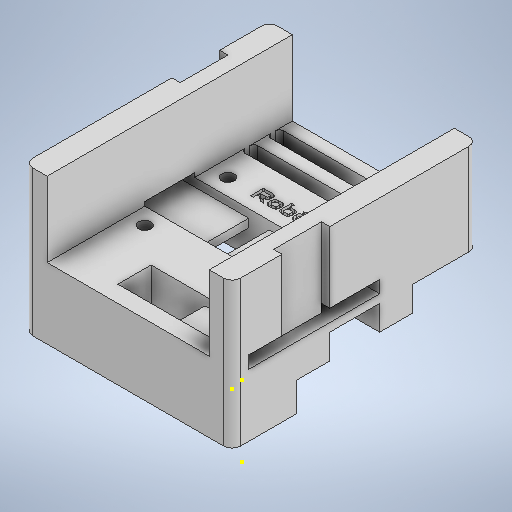
# Autodesk Inventor part: CaseInterno
Saved by Autodesk Inventor 2025.2 (Build 292293000, 293)
## iProperties
Created: 2025-03-20
Part Number: CaseInterno
Material: Genérico
Document SubType Name: Modeling
Designer: miche
Density: 1 g/cm^3
Appearance: Padrão
Author: miche
Autodesk Inventor part; units mm, degrees
ref_plane "YZ Plane" through (0, 0, 0) normal (1, 0, 0) x (0, 1, 0)
ref_plane "XZ Plane" through (0, 0, 0) normal (0, 1, 0) x (-1, 0, 0)
ref_plane "XY Plane" through (0, 0, 0) normal (0, 0, 1) x (1, 0, 0)
sketch "Esboço1" plane through (0, 0, 0) normal (0, 1, 0) x (-1, 0, 0)
  line L0 (5, 0) -> (50, 0)
  line L1 (55, -5) -> (55, -54)
  line L2 (50, -59) -> (5, -59)
  line L3 (0, -54) -> (0, -5)
  arc A0 (50, -59) -> (55, -54) centre (50, -54) ccw
  arc A1 (0, -54) -> (5, -59) centre (5, -54) ccw
  arc A2 (5, 0) -> (0, -5) centre (5, -5) ccw
  arc A3 (55, -5) -> (50, 0) centre (50, -5) ccw
  point P0 (0, 0)
  point P1 (55, -59)
  point P2 (55, 0)
  point P3 (0, -59)
  dimension "d0" = 55
  dimension "d1" = 59
  dimension "d2" = 5
  constraints: 8 end point, 8 point on circle, 8 point on line, 8 tangent, 4 centre point, 3 equal radius, 2 parallel, 1 horizontal, 1 perpendicular
  measures "d0" distance of point (55, -59) point (0, -59)
  measures "d1" distance of point (55, 0) point (55, -59)
  measures "d2" radius of A0
extrude "Extrusão1" add sketch "Esboço1" along normal blind 5
sketch "Esboço2" plane through (0, 0, 0) normal (0, -1, 0) x (1, 0, 0)
  line L0 (-5, -59) -> (-50, -59) projected
  line L1 (-50, -59) -> (-55, -59)
  arc A0 (-55, -54) -> (-50, -59) centre (-50, -54) ccw projected
  line L2 (-55, -59) -> (-55, -43.5)
  line L3 (-55, -54) -> (-55, -5) projected
  line L4 (-55, -5) -> (-55, 0)
  line L5 (-55, 0) -> (-50, 0)
  line L6 (-55, 0) -> (-55, -15.5)
  line L7 (0, -5) -> (0, -54) projected
  line L8 (-55, -43.5) -> (0, -43.5)
  line L9 (0, -43.5) -> (0, -35.5)
  line L10 (0, -35.5) -> (-55, -35.5)
  line L11 (-55, -35.5) -> (-55, -43.5)
  line L12 (-55, -15.5) -> (0, -15.5)
  line L13 (0, -15.5) -> (0, -23.5)
  line L14 (0, -23.5) -> (-55, -23.5)
  line L15 (-55, -23.5) -> (-55, -15.5)
  line L16 (-55, -35.5) -> (-55, -23.5)
  line L17 (0, -35.5) -> (0, -23.5)
  point P0 (0, 0)
  dimension "d5" = 15.5
  dimension "d6" = 15.5
  dimension "d7" = 8
  dimension "d8" = 8
  constraints: 30 end point, 4 parallel, 4 point on line, 3 horizontal, 3 perpendicular, 1 collinear, 1 tangent, 1 vertical
  measures "d5" distance of L1.end L2.end
  measures "d6" distance of L4.end L6.end
  measures "d7" distance of L9.end L8.end
  measures "d8" distance of L12.end L13.end
extrude "Extrusão2" add sketch "Esboço2" along normal blind 6 contours L3 L10 L7 L8 | L3 L12 L7 L14
sketch "Esboço3" plane through (0, -6, 0) normal (0, -1, 0) x (1, 0, 0)
  line L0 (-55, -43.5) -> (0, -43.5) projected
  line L1 (-55, -35.5) -> (0, -35.5) projected
  line L2 (0, -43.5) -> (-24, -43.5)
  line L3 (-24, -43.5) -> (-24, -35.5)
  line L4 (-24, -35.5) -> (0, -35.5)
  line L5 (0, -35.5) -> (0, -43.5)
  line L6 (-55, -35.5) -> (-55, -43.5) projected
  line L7 (-55, -43.5) -> (-31, -43.5)
  line L8 (-31, -43.5) -> (-31, -35.5)
  line L9 (-31, -35.5) -> (-55, -35.5)
  line L10 (-55, -35.5) -> (-55, -43.5)
  line L11 (-24, -43.5) -> (-31, -43.5)
  line L12 (-31, -43.5) -> (-31, -35.5)
  line L13 (-31, -35.5) -> (-24, -35.5)
  line L14 (-24, -35.5) -> (-24, -43.5)
  line L15 (-55, -15.5) -> (0, -15.5) projected
  line L16 (0, -23.5) -> (-55, -23.5) projected
  line L17 (0, -15.5) -> (-24, -15.5)
  line L18 (-24, -15.5) -> (-24, -23.5)
  line L19 (-24, -23.5) -> (0, -23.5)
  line L20 (0, -23.5) -> (0, -15.5)
  line L21 (-24, -23.5) -> (-31, -23.5)
  line L22 (-31, -23.5) -> (-31, -15.5)
  line L23 (-31, -15.5) -> (-24, -15.5)
  line L24 (-24, -15.5) -> (-24, -23.5)
  point P0 (0, 0)
  constraints: 40 end point, 10 parallel, 6 point on line, 5 horizontal, 5 perpendicular
extrude "Extrusão3" add sketch "Esboço3" along normal blind 16 contours L8 L1 L3 L0 | L15 L18 L16 L22
sketch "Esboço4" plane through (0, -6, 0) normal (0, -1, 0) x (1, 0, 0)
  line L0 (0, -43.5) -> (-55, -43.5) projected
  line L1 (0, -43.5) -> (-12, -43.5)
  line L2 (-12, -43.5) -> (-12, -39.5)
  line L3 (-55, -43.5) -> (-43, -43.5)
  line L4 (-55, -43.5) -> (-31, -43.5) projected
  line L5 (-43, -43.5) -> (-43, -39.5)
  line L6 (-55, -15.5) -> (0, -15.5) projected
  line L7 (0, -15.5) -> (-12, -15.5)
  line L8 (-12, -15.5) -> (-12, -19.5)
  line L9 (-55, -15.5) -> (-43, -15.5)
  line L10 (-55, -15.5) -> (-43, -15.5)
  line L11 (-43, -15.5) -> (-43, -19.5)
  circle A0 centre (-12, -39.5) radius 1.5
  circle A1 centre (-12, -19.5) radius 1.5
  circle A2 centre (-43, -39.5) radius 1.5
  circle A3 centre (-43, -19.5) radius 1.5
  point P0 (0, 0)
  dimension "d13" = 4
  dimension "d14" = 12
  dimension "d15" = 4
  dimension "d16" = 12
  dimension "d17" = 4
  dimension "d18" = 12
  dimension "d19" = 4
  dimension "d20" = 3
  dimension "d21" = 3
  dimension "d22" = 3
  dimension "d23" = 3
  constraints: 18 end point, 4 centre point, 4 coincident, 3 perpendicular, 3 point on line, 1 collinear, 1 midpoint, 1 vertical
  measures "d13" distance of L1.end L2.end
  measures "d14" distance of L0.end L3.end
  measures "d15" distance of L3.end L5.end
  measures "d16" distance of L6.end L7.end
  measures "d17" distance of L7.end L8.end
  measures "d18" distance of L6.start L9.end
  measures "d19" distance of L9.end L11.end
  measures "d20" diameter of A0
  measures "d21" diameter of A1
  measures "d22" diameter of A2
  measures "d23" diameter of A3
extrude "Extrusão4" cut sketch "Esboço4" against normal blind 11
thread "Rosca1" size "M3x0.5" class "6H" standard "ANSI Metric M Profile" length 11
thread "Rosca2" size "M3x0.5" class "6H" standard "ANSI Metric M Profile" full length
thread "Rosca3" size "M3x0.5" class "6H" standard "ANSI Metric M Profile" full length
thread "Rosca4" size "M3x0.5" class "6H" standard "ANSI Metric M Profile" full length
thread "Rosca5" size "M3x0.5" class "6H" standard "ANSI Metric M Profile" length 11
thread "Rosca6" size "M3x0.5" class "6H" standard "ANSI Metric M Profile" length 11
thread "Rosca7" size "M3x0.5" class "6H" standard "ANSI Metric M Profile" length 11
sketch "Esboço7" plane through (0, 0, 0) normal (0, -1, 0) x (1, 0, 0)
  line L0 (-55, -35.5) -> (0, -35.5) projected
  line L1 (0, -35.5) -> (-24, -35.5)
  line L2 (-31, -23.5) -> (-31, -15.5) projected
  line L3 (-24, -35.5) -> (-31, -35.5)
  line L4 (-31, -35.5) -> (-31, -23.5)
  line L5 (-31, -23.5) -> (-24, -23.5)
  line L6 (-24, -23.5) -> (-24, -35.5)
  point P0 (0, 0)
  constraints: 10 end point, 2 parallel, 1 horizontal, 1 perpendicular, 1 point on line
extrude "Extrusão7" add sketch "Esboço7" along normal blind 6
sketch "Esboço9" plane through (0, 0, 0) normal (0, -1, 0) x (1, 0, 0)
  line L0 (0, -5) -> (0, -15.5) projected
  line L1 (0, -15.5) -> (0, -5)
  line L2 (-50, 0) -> (-5, 0) projected
  arc A0 (0, -5) -> (-5, 0) centre (-5, -5) ccw
  line L3 (-55, -15.5) -> (0, -15.5) projected
  line L4 (-55, -15.5) -> (-55, -5)
  arc A1 (-50, 0) -> (-55, -5) centre (-50, -5) ccw projected
  line L5 (-5, 0) -> (-50, 0)
  arc A2 (-50, 0) -> (-55, -5) centre (-50, -5) ccw
  point P0 (0, 0)
  constraints: 6 end point, 4 point on circle, 2 centre point, 2 tangent, 1 collinear, 1 horizontal
sketch "Esboço10" plane through (0, 0, 0) normal (0, -1, 0) x (1, 0, 0)
  line L0 (-24, -35.5) -> (-24, -23.5) projected
  line L1 (-24, -23.5) -> (0, -23.5) projected
  line L2 (-24, -35.5) -> (-21, -35.5)
  line L3 (-21, -35.5) -> (-21, -23.5)
  line L4 (-21, -23.5) -> (-24, -23.5)
  line L5 (-24, -23.5) -> (-24, -35.5)
  line L6 (-31, -23.5) -> (-31, -35.5) projected
  line L7 (-31, -35.5) -> (-34, -35.5)
  line L8 (-34, -35.5) -> (-34, -23.5)
  line L9 (-34, -23.5) -> (-31, -23.5)
  line L10 (-31, -23.5) -> (-31, -35.5)
  point P0 (0, 0)
  constraints: 16 end point, 4 parallel, 2 horizontal, 2 perpendicular, 2 point on line
extrude "Extrusão9" cut sketch "Esboço10" against normal through all
sketch "Esboço11" plane through (0, 5, 0) normal (0, 1, 0) x (1, 0, 0)
  line L0 (-34, 23.5) -> (-34, 35.5)
  line L1 (-24, 23.5) -> (-24, 35.5) projected
  line L2 (-31, 23.5) -> (-31, 35.5) projected
  line L3 (-24, 35.5) -> (-31, 35.5)
  line L4 (-31, 35.5) -> (-31, 23.5)
  line L5 (-31, 23.5) -> (-24, 23.5)
  line L6 (-24, 23.5) -> (-24, 35.5)
  line L7 (-21, 35.5) -> (0, 35.5) projected
  line L8 (0, 23.5) -> (-21, 23.5) projected
  line L9 (-21, 35.5) -> (-2, 35.5)
  line L10 (-2, 23.5) -> (-21, 23.5)
  line L11 (-21, 23.5) -> (-21, 35.5)
  line L12 (-2, 35.5) -> (0, 35.5)
  line L13 (0, 35.5) -> (0, 23.5)
  line L14 (0, 23.5) -> (-2, 23.5)
  line L15 (-2, 23.5) -> (-2, 35.5)
  point P0 (0, 0)
  constraints: 24 end point, 5 parallel, 3 horizontal, 2 perpendicular, 1 point on line
extrude "Extrusão10" cut sketch "Esboço11" against normal blind 2
extrude "Extrusão11" add sketch "Esboço9" along normal blind 13
sketch "Esboço12" plane through (0, -13, 0) normal (0, -1, 0) x (1, 0, 0)
  line L0 (-9.5, 0) -> (-5, 0) projected
  line L1 (-5, 0) -> (-5, -15.5)
  line L2 (-5, -23.5) -> (-5, 0) projected
  line L3 (0, -15.5) -> (-24, -15.5) projected
  line L4 (0, -15.5) -> (-55, -15.5)
  line L5 (0, -15.5) -> (-20, -15.5)
  line L6 (-20, -15.5) -> (-12.7, -15.5) construction
  line L7 (-20, -13) -> (-35, -13)
  line L8 (-35, -13) -> (-35, -3)
  line L9 (-35, -3) -> (-20, -3)
  line L10 (-20, -3) -> (-20, -13)
  point P0 (0, 0)
  constraints: 16 end point, 3 horizontal, 2 parallel, 2 point on line, 1 perpendicular
extrude "Extrusão12" cut sketch "Esboço12" against normal blind 1
sketch "Esboço13" plane through (0, -12, 0) normal (0, -1, 0) x (1, 0, 0)
  line L0 (-35, -13) -> (-35, -3) projected
  line L1 (-35, -3) -> (-34, -3)
  line L2 (-35, -3) -> (-20, -3) projected
  line L3 (-34, -3) -> (-34, -4)
  line L4 (-34, -4) -> (-21, -4)
  line L5 (-21, -4) -> (-21, -12)
  line L6 (-21, -12) -> (-34, -12)
  line L7 (-34, -12) -> (-34, -4)
  point P0 (0, 0)
  constraints: 12 end point, 2 parallel, 1 horizontal, 1 perpendicular, 1 point on line, 1 vertical
extrude "Extrusão13" cut sketch "Esboço13" against normal blind 16
sketch "Esboço14" plane through (0, 5, 0) normal (0, 1, 0) x (1, 0, 0)
  line L0 (-21, 12) -> (-34, 12) projected
  line L1 (-34, 12) -> (-21, 12)
  line L2 (-21, 12) -> (-21, 4)
  line L3 (-21, 4) -> (-34, 4)
  line L4 (-34, 4) -> (-34, 12)
  line L5 (-21, 12) -> (-2, 12)
  line L6 (-2, 4) -> (-21, 4)
  line L7 (-21, 4) -> (-21, 12) projected
  line L8 (-21, 12) -> (-21, 4)
  line L9 (-2, 12) -> (0, 12)
  line L10 (0, 12) -> (0, 4)
  line L11 (0, 4) -> (-2, 4)
  line L12 (-2, 4) -> (-2, 12)
  point P0 (0, 0)
  constraints: 22 end point, 4 perpendicular, 3 equal length, 1 horizontal, 1 point on line, 1 vertical
extrude "Extrusão14" cut sketch "Esboço14" against normal blind 2
sketch "Esboço16" plane through (0, 5, 0) normal (0, 1, 0) x (1, 0, 0)
  arc A0 (-50, 59) -> (-55, 54) centre (-50, 54) ccw projected
  line L0 (-55, 54) -> (-55, 5) projected
  line L1 (-55, 54) -> (-55, 5)
  line L2 (-55, 5) -> (-47, 5)
  line L3 (-47, 5) -> (-47, 54)
  line L4 (-47, 54) -> (-55, 54)
  line L5 (-47, 5) -> (-47, 0)
  line L6 (-47, 54) -> (-47, 59)
  line L7 (-5, 59) -> (-50, 59) projected
  arc A1 (-50, 59) -> (-55, 54) centre (-50, 54) ccw
  arc A2 (-55, 5) -> (-50, 0) centre (-50, 5) ccw
  arc A3 (0, 54) -> (-5, 59) centre (-5, 54) ccw projected
  arc A4 (0, 54) -> (-5, 59) centre (-5, 54) ccw
  arc A5 (-5, 0) -> (0, 5) centre (-5, 5) ccw projected
  arc A6 (-5, 0) -> (0, 5) centre (-5, 5) ccw
  line L8 (0, 43.5) -> (0, 54) projected
  line L9 (0, 54) -> (0, 5)
  line L10 (0, 54) -> (-8, 54)
  line L11 (-8, 54) -> (-8, 59)
  line L12 (-8, 54) -> (-8, 4)
  line L13 (-0.101, 4) -> (-21, 4) projected
  line L14 (-5, 0) -> (-50, 0) projected
  line L15 (-8, 0) -> (-5, 0)
  line L16 (-8, 4) -> (-8, 0)
  point P0 (0, 0)
  constraints: 24 end point, 8 point on circle, 6 point on line, 5 tangent, 4 centre point, 3 collinear, 3 perpendicular, 3 vertical, 1 horizontal
extrude "Extrusão15" add sketch "Esboço16" along normal blind 17 contours L7 L6 L4 A0 | L4 L3 L2 L0 | L2 L5 L14 A2 | L7 A3 L10 L11 | L10 L8 L9 A5 L13 L12 | L13 A5 L14 L16
sketch "Esboço20" plane through (0, 0, 0) normal (0, -1, 0) x (1, 0, 0)
  arc A0 (-5, -59) -> (0, -54) centre (-5, -54) ccw projected
  line L0 (-9, -55.9) -> (-46, -55.9)
  line L1 (-8, -55.9) -> (-47, -55.9)
  line L2 (-47, -54.9) -> (-47, -53.8)
  line L3 (-46, -52.8) -> (-9, -52.8)
  line L4 (-8, -53.8) -> (-8, -54.9)
  line L5 (-8, -52.8) -> (-47, -52.8)
  line L6 (-47, -49.7) -> (-9, -49.7)
  line L7 (-8, -49.7) -> (-46, -49.7)
  line L8 (-47, -48.7) -> (-47, -47.6)
  line L9 (-46, -46.6) -> (-9, -46.6)
  line L10 (-8, -47.6) -> (-8, -48.7)
  arc A1 (-9, -55.9) -> (-8, -54.9) centre (-9, -54.9) ccw
  arc A2 (-8, -53.8) -> (-9, -52.8) centre (-9, -53.8) ccw
  arc A3 (-47, -54.9) -> (-46, -55.9) centre (-46, -54.9) ccw
  arc A4 (-46, -52.8) -> (-47, -53.8) centre (-46, -53.8) ccw
  arc A5 (-9, -49.7) -> (-8, -48.7) centre (-9, -48.7) ccw
  arc A6 (-8, -47.6) -> (-9, -46.6) centre (-9, -47.6) ccw
  arc A7 (-46, -46.6) -> (-47, -47.6) centre (-46, -47.6) ccw
  arc A8 (-47, -48.7) -> (-46, -49.7) centre (-46, -48.7) ccw
  point P0 (0, 0)
  dimension "d97" = 1
  constraints: 22 end point, 16 point on circle, 16 tangent, 8 centre point, 7 equal radius, 7 point on line, 5 parallel, 3 horizontal, 2 perpendicular
  measures "d97" radius of A1
extrude "Extrusão18" cut sketch "Esboço20" against normal through all
sketch "Esboço22" plane through (0, 5, 0) normal (0, 1, 0) x (1, 0, 0)
  line L0 (-39.1857, 44.1197) -> (-14.6747, 44.1197) construction
  line L1 (-14.6747, 44.1197) -> (-14.6747, 36.2889) construction
  line L2 (-14.6747, 36.2889) -> (-39.1857, 36.2889) construction
  line L3 (-39.1857, 36.2889) -> (-39.1857, 44.1197) construction
  spline S0 degree 2 poles (-33.3948, 40.4658) (-33.3948, 40.2734) (-33.4897, 39.97) (-33.6549, 39.7342) (-33.8663, 39.569) (-34.0993, 39.4633) (-34.335, 39.4145) (-34.3946, 39.4145) knots 0 0 0 1 2 3 4 5 6 6 6
  line L4 (-34.3946, 39.4145) -> (-33.2648, 38.4392)
  line L5 (-33.2648, 38.4392) -> (-34.1643, 38.4392)
  line L6 (-34.1643, 38.4392) -> (-35.2941, 39.4145)
  line L7 (-35.2941, 39.4145) -> (-35.7087, 39.4145)
  line L8 (-35.7087, 39.4145) -> (-35.7087, 40.0431)
  line L9 (-35.7087, 40.0431) -> (-34.438, 40.0431)
  spline S1 degree 2 poles (-34.438, 40.0431) (-34.3513, 40.0512) (-34.1941, 40.1136) (-34.0857, 40.2192) (-34.0234, 40.3682) (-34.0234, 40.4658) knots 0 0 0 1 2 3 4 4 4
  line L10 (-34.0234, 40.4658) -> (-34.0234, 40.8072)
  spline S2 degree 2 poles (-34.0234, 40.8072) (-34.0234, 40.8424) (-34.037, 40.8695) (-34.0532, 40.8803) (-34.083, 40.883) (-34.0966, 40.883) knots 0 0 0 1 2 3 4 4 4
  line L11 (-34.0966, 40.883) -> (-35.836, 40.883)
  line L12 (-35.836, 40.883) -> (-35.836, 38.4392)
  line L13 (-35.836, 38.4392) -> (-36.4673, 38.4392)
  line L14 (-36.4673, 38.4392) -> (-36.4673, 41.1946)
  spline S3 degree 2 poles (-36.4673, 41.1946) (-36.4673, 41.2623) (-36.4212, 41.3761) (-36.3345, 41.4628) (-36.218, 41.5116) (-36.1503, 41.5116) knots 0 0 0 1 2 3 4 4 4
  line L15 (-36.1503, 41.5116) -> (-34.0966, 41.5116)
  spline S4 degree 2 poles (-34.0966, 41.5116) (-33.9042, 41.5116) (-33.6333, 41.3707) (-33.468, 41.1594) (-33.3948, 40.9155) (-33.3948, 40.8099) knots 0 0 0 1 2 3 4 4 4
  line L16 (-33.3948, 40.8099) -> (-33.3948, 40.4658)
  spline S5 degree 2 poles (-30.3847, 39.2438) (-30.3847, 39.0975) (-30.4606, 38.8618) (-30.5852, 38.683) (-30.7478, 38.5557) (-30.9266, 38.4771) (-31.1108, 38.4392) (-31.1921, 38.4392) knots 0 0 0 1 2 3 4 5 6 6 6
  line L17 (-31.1921, 38.4392) -> (-32.1675, 38.4392)
  spline S6 degree 2 poles (-32.1675, 38.4392) (-32.2894, 38.4392) (-32.5685, 38.5231) (-32.8096, 38.7128) (-32.9695, 39.0217) (-32.9695, 39.2438) knots 0 0 0 1 2 3 4 4 4
  line L18 (-32.9695, 39.2438) -> (-32.9695, 39.9754)
  spline S7 degree 2 poles (-32.9695, 39.9754) (-32.9695, 40.1948) (-32.8096, 40.501) (-32.5685, 40.6934) (-32.2867, 40.7774) (-32.1675, 40.7774) knots 0 0 0 1 2 3 4 4 4
  line L19 (-32.1675, 40.7774) -> (-31.1921, 40.7774)
  spline S8 degree 2 poles (-31.1921, 40.7774) (-30.9726, 40.7774) (-30.6611, 40.6175) (-30.4714, 40.3764) (-30.3847, 40.0946) (-30.3847, 39.9754) knots 0 0 0 1 2 3 4 4 4
  line L20 (-30.3847, 39.9754) -> (-30.3847, 39.2438)
  spline S9 degree 2 poles (-31.016, 39.9727) (-31.016, 40.0648) (-31.1054, 40.1488) (-31.1921, 40.1488) knots 0 0 0 1 2 2 2
  line L21 (-31.1921, 40.1488) -> (-32.1648, 40.1488)
  spline S10 degree 2 poles (-32.1648, 40.1488) (-32.2542, 40.1488) (-32.3382, 40.0648) (-32.3382, 39.9754) knots 0 0 0 1 2 2 2
  line L22 (-32.3382, 39.9754) -> (-32.3382, 39.2438)
  spline S11 degree 2 poles (-32.3382, 39.2438) (-32.3382, 39.1544) (-32.2542, 39.0677) (-32.1648, 39.0677) knots 0 0 0 1 2 2 2
  line L23 (-32.1648, 39.0677) -> (-31.1921, 39.0677)
  spline S12 degree 2 poles (-31.1921, 39.0677) (-31.1, 39.0677) (-31.016, 39.1544) (-31.016, 39.2438) knots 0 0 0 1 2 2 2
  line L24 (-31.016, 39.2438) -> (-31.016, 39.9727)
  spline S13 degree 2 poles (-27.38, 39.2438) (-27.38, 39.1626) (-27.4179, 38.981) (-27.4965, 38.8049) (-27.6211, 38.6424) (-27.8026, 38.515) (-28.0384, 38.4392) (-28.1847, 38.4392) knots 0 0 0 1 2 3 4 5 6 6 6
  line L25 (-28.1847, 38.4392) -> (-29.1601, 38.4392)
  spline S14 degree 2 poles (-29.1601, 38.4392) (-29.244, 38.4392) (-29.4229, 38.4771) (-29.6017, 38.5557) (-29.7642, 38.6803) (-29.8889, 38.8591) (-29.9647, 39.0948) (-29.9647, 39.2438) knots 0 0 0 1 2 3 4 5 6 6 6
  line L26 (-29.9647, 39.2438) -> (-29.9647, 41.7284)
  line L27 (-29.9647, 41.7284) -> (-29.3335, 41.7284)
  line L28 (-29.3335, 41.7284) -> (-29.3335, 39.2438)
  spline S15 degree 2 poles (-29.3335, 39.2438) (-29.3335, 39.1599) (-29.2359, 39.0677) (-29.1601, 39.0677) knots 0 0 0 1 2 2 2
  line L29 (-29.1601, 39.0677) -> (-28.1847, 39.0677)
  spline S16 degree 2 poles (-28.1847, 39.0677) (-28.1007, 39.0677) (-28.0113, 39.1626) (-28.0113, 39.2438) knots 0 0 0 1 2 2 2
  line L30 (-28.0113, 39.2438) -> (-28.0113, 39.9754)
  spline S17 degree 2 poles (-28.0113, 39.9754) (-28.0113, 40.0567) (-28.1061, 40.1488) (-28.1847, 40.1488) knots 0 0 0 1 2 2 2
  line L31 (-28.1847, 40.1488) -> (-29.2034, 40.1488)
  line L32 (-29.2034, 40.1488) -> (-29.2034, 40.7774)
  line L33 (-29.2034, 40.7774) -> (-28.1847, 40.7774)
  spline S18 degree 2 poles (-28.1847, 40.7774) (-28.1061, 40.7774) (-27.9219, 40.7394) (-27.743, 40.6582) (-27.5805, 40.5335) (-27.4558, 40.3547) (-27.38, 40.119) (-27.38, 39.9754) knots 0 0 0 1 2 3 4 5 6 6 6
  line L34 (-27.38, 39.9754) -> (-27.38, 39.2438)
  spline S19 degree 2 poles (-24.4051, 39.2438) (-24.4051, 39.0975) (-24.4809, 38.8618) (-24.6055, 38.683) (-24.7681, 38.5557) (-24.9469, 38.4771) (-25.1312, 38.4392) (-25.2125, 38.4392) knots 0 0 0 1 2 3 4 5 6 6 6
  line L35 (-25.2125, 38.4392) -> (-26.1878, 38.4392)
  spline S20 degree 2 poles (-26.1878, 38.4392) (-26.3098, 38.4392) (-26.5888, 38.5231) (-26.83, 38.7128) (-26.9898, 39.0217) (-26.9898, 39.2438) knots 0 0 0 1 2 3 4 4 4
  line L36 (-26.9898, 39.2438) -> (-26.9898, 39.9754)
  spline S21 degree 2 poles (-26.9898, 39.9754) (-26.9898, 40.1948) (-26.83, 40.501) (-26.5888, 40.6934) (-26.3071, 40.7774) (-26.1878, 40.7774) knots 0 0 0 1 2 3 4 4 4
  line L37 (-26.1878, 40.7774) -> (-25.2125, 40.7774)
  spline S22 degree 2 poles (-25.2125, 40.7774) (-24.993, 40.7774) (-24.6814, 40.6175) (-24.4918, 40.3764) (-24.4051, 40.0946) (-24.4051, 39.9754) knots 0 0 0 1 2 3 4 4 4
  line L38 (-24.4051, 39.9754) -> (-24.4051, 39.2438)
  spline S23 degree 2 poles (-25.0363, 39.9727) (-25.0363, 40.0648) (-25.1258, 40.1488) (-25.2125, 40.1488) knots 0 0 0 1 2 2 2
  line L39 (-25.2125, 40.1488) -> (-26.1851, 40.1488)
  spline S24 degree 2 poles (-26.1851, 40.1488) (-26.2745, 40.1488) (-26.3585, 40.0648) (-26.3585, 39.9754) knots 0 0 0 1 2 2 2
  line L40 (-26.3585, 39.9754) -> (-26.3585, 39.2438)
  spline S25 degree 2 poles (-26.3585, 39.2438) (-26.3585, 39.1544) (-26.2745, 39.0677) (-26.1851, 39.0677) knots 0 0 0 1 2 2 2
  line L41 (-26.1851, 39.0677) -> (-25.2125, 39.0677)
  spline S26 degree 2 poles (-25.2125, 39.0677) (-25.1203, 39.0677) (-25.0363, 39.1544) (-25.0363, 39.2438) knots 0 0 0 1 2 2 2
  line L42 (-25.0363, 39.2438) -> (-25.0363, 39.9727)
  line L43 (-24.9605, 40.9806) -> (-25.7001, 41.3545)
  line L44 (-25.7001, 41.3545) -> (-26.4371, 40.9806)
  line L45 (-26.4371, 40.9806) -> (-26.7216, 41.387)
  line L46 (-26.7216, 41.387) -> (-25.7001, 41.9695)
  line L47 (-25.7001, 41.9695) -> (-24.6787, 41.387)
  line L48 (-24.6787, 41.387) -> (-24.9605, 40.9806)
  line L49 (-20.8937, 38.4392) -> (-21.5222, 38.4392)
  line L50 (-21.5222, 38.4392) -> (-21.5222, 39.1734)
  line L51 (-21.5222, 39.1734) -> (-23.3375, 39.1734)
  line L52 (-23.3375, 39.1734) -> (-23.3375, 38.4392)
  line L53 (-23.3375, 38.4392) -> (-23.9688, 38.4392)
  line L54 (-23.9688, 38.4392) -> (-23.9688, 39.9754)
  spline S27 degree 2 poles (-23.9688, 39.9754) (-23.9688, 40.3113) (-23.7358, 40.8776) (-23.324, 41.284) (-22.7632, 41.5116) (-22.4326, 41.5116) knots 0 0 0 1 2 3 4 4 4
  line L55 (-22.4326, 41.5116) -> (-21.2107, 41.5116)
  spline S28 degree 2 poles (-21.2107, 41.5116) (-21.1456, 41.5116) (-21.0291, 41.4628) (-20.9397, 41.3761) (-20.8937, 41.2596) (-20.8937, 41.1946) knots 0 0 0 1 2 3 4 4 4
  line L56 (-20.8937, 41.1946) -> (-20.8937, 38.4392)
  line L57 (-23.3375, 39.7993) -> (-21.5222, 39.7993)
  line L58 (-21.5222, 39.7993) -> (-21.5222, 40.883)
  line L59 (-21.5222, 40.883) -> (-22.4326, 40.883)
  spline S29 degree 2 poles (-22.4326, 40.883) (-22.4543, 40.883) (-22.6087, 40.8695) (-22.8092, 40.8126) (-23.0314, 40.6988) (-23.2156, 40.4983) (-23.3375, 40.1948) (-23.3375, 39.9754) knots 0 0 0 1 2 3 4 5 6 6 6
  line L60 (-23.3375, 39.9754) -> (-23.3375, 39.7993)
  spline S30 degree 2 poles (-17.2116, 40.2192) (-17.2116, 40.0269) (-17.3064, 39.7234) (-17.4717, 39.4904) (-17.683, 39.3251) (-17.916, 39.2195) (-18.1545, 39.1734) (-18.2574, 39.1734) knots 0 0 0 1 2 3 4 5 6 6 6
  line L61 (-18.2574, 39.1734) -> (-19.5254, 39.1734)
  line L62 (-19.5254, 39.1734) -> (-19.5254, 39.7993)
  line L63 (-19.5254, 39.7993) -> (-18.2547, 39.7993)
  spline S31 degree 2 poles (-18.2547, 39.7993) (-18.1653, 39.8074) (-18.0109, 39.8697) (-17.9025, 39.9754) (-17.8402, 40.1244) (-17.8402, 40.2192) knots 0 0 0 1 2 3 4 4 4
  line L64 (-17.8402, 40.2192) -> (-17.8402, 40.4604)
  spline S32 degree 2 poles (-17.8402, 40.4604) (-17.851, 40.5552) (-17.9133, 40.7123) (-18.0163, 40.8234) (-18.1599, 40.883) (-18.2574, 40.883) knots 0 0 0 1 2 3 4 4 4
  line L65 (-18.2574, 40.883) -> (-19.4794, 40.883)
  spline S33 degree 2 poles (-19.4794, 40.883) (-19.5661, 40.883) (-19.6528, 40.7963) (-19.6528, 40.7096) knots 0 0 0 1 2 2 2
  line L66 (-19.6528, 40.7096) -> (-19.6528, 38.4392)
  line L67 (-19.6528, 38.4392) -> (-20.2841, 38.4392)
  line L68 (-20.2841, 38.4392) -> (-20.2841, 40.7096)
  spline S34 degree 2 poles (-20.2841, 40.7096) (-20.2841, 40.9264) (-20.1215, 41.238) (-19.8831, 41.4276) (-19.6013, 41.5116) (-19.4821, 41.5116) knots 0 0 0 1 2 3 4 4 4
  line L69 (-19.4821, 41.5116) -> (-18.2574, 41.5116)
  spline S35 degree 2 poles (-18.2574, 41.5116) (-18.0705, 41.5116) (-17.7616, 41.4141) (-17.5286, 41.2488) (-17.3633, 41.0348) (-17.2604, 40.8045) (-17.2116, 40.566) (-17.2116, 40.4658) knots 0 0 0 1 2 3 4 5 6 6 6
  line L70 (-17.2116, 40.4658) -> (-17.2116, 40.2192)
  point P0 (0, 0)
  constraints: 2 other
extrude "Extrusão20" cut sketch "Esboço22" against normal blind 2
sketch "Esboço24" plane through (0, 22, 0) normal (0, 1, 0) x (1, 0, 0)
  arc A0 (-50, 59) -> (-55, 54) centre (-50, 54) ccw projected
  line L0 (-55, 54) -> (-55, 59)
  line L1 (-55, 59) -> (-50, 59)
  arc A1 (-50, 59) -> (-55, 54) centre (-50, 54) ccw
  arc A2 (0, 54) -> (-5, 59) centre (-5, 54) ccw projected
  line L2 (-5, 59) -> (-50, 59) projected
  arc A3 (0, 54) -> (-5, 59) centre (-5, 54) ccw
  arc A4 (-55, 5) -> (-50, 0) centre (-50, 5) ccw projected
  arc A5 (-55, 5) -> (-50, 0) centre (-50, 5) ccw
  arc A6 (-5, 0) -> (0, 5) centre (-5, 5) ccw projected
  line L3 (-0.101, 4) -> (-21, 4) projected
  arc A7 (-5, 0) -> (-0.101, 4) centre (-5, 5) ccw
  line L4 (0, 54) -> (0, 59)
  line L5 (0, 59) -> (-5, 59)
  arc A8 (-0.101, 4) -> (0, 5) centre (-5, 5) ccw projected
  line L6 (0, 5) -> (0, 0)
  line L7 (0, 0) -> (-5, 0)
  line L8 (-55, 5) -> (-55, 0)
  line L9 (-55, 0) -> (-50, 0)
  constraints: 16 end point, 11 tangent, 9 point on circle, 4 centre point, 4 perpendicular, 3 vertical
extrude "Extrusão22" add sketch "Esboço24" against normal blind 36 contours A4 L9 L8 | A6 L6 L7
extrude "Extrusão23" add sketch "Esboço24" against normal blind 23 contours A0 L0 L1 | L5 L4 A2
sketch "Esboço25" plane through (0, 22, 0) normal (0, 1, 0) x (1, 0, 0)
  line L0 (-47, 0) -> (-47, 59) projected
  line L1 (-8, 59) -> (-8, 0) projected
  line L2 (-47, 59) -> (-8, 59)
  line L3 (0, 0) -> (-55, 0) projected
  line L4 (-8, 59) -> (-2.5, 59)
  line L5 (-2.5, 59) -> (-2.5, 0)
  line L6 (-2.5, 0) -> (-8, 0)
  line L7 (-8, 0) -> (-8, 59)
  line L8 (0, 0) -> (0, 59) projected
  line L9 (-2.5, 59) -> (0, 59)
  line L10 (0, 59) -> (0, 0)
  line L11 (0, 0) -> (-2.5, 0)
  line L12 (-2.5, 0) -> (-2.5, 59)
  line L13 (-47, 59) -> (-52.5, 59)
  line L14 (-52.5, 59) -> (-52.5, 0)
  line L15 (-52.5, 0) -> (-47, 0)
  line L16 (-47, 0) -> (-47, 59)
  line L17 (-55, 0) -> (-55, 15.5) projected
  line L18 (-52.5, 59) -> (-55, 59)
  line L19 (-55, 59) -> (-55, 0)
  line L20 (-55, 0) -> (-52.5, 0)
  line L21 (-52.5, 0) -> (-52.5, 59)
  dimension "d125" = 5.5
  dimension "d126" = 5.5
  dimension "d127" = 59
  constraints: 34 end point, 8 parallel, 5 horizontal, 4 perpendicular, 1 point on line
  measures "d125" distance of L5.end L6.end
  measures "d126" distance of L15.end L14.end
  measures "d127" distance of L14.end L13.end
extrude "Extrusão24" cut sketch "Esboço25" against normal through all contours L3 L17 L19 L18 L14 | L5 L9 L8 L3
sketch "Esboço26" plane through (-2.5, 22, 0) normal (1, 0, 0) x (0, 0, -1)
  point P0 (0, -22)
sketch "Esboço27" plane through (-2.5, 22, 0) normal (1, 0, 0) x (0, 0, -1)
  line L0 (23.5, -17) -> (23.5, -19) projected
  line L1 (23.5, -17) -> (12, -17)
  line L2 (12, -17) -> (12, 1)
  line L3 (12, 1) -> (23.5, 1)
  line L4 (23.5, 1) -> (23.5, -17)
  line L5 (23.5, -17) -> (12, -17)
  line L6 (12, -17) -> (12, -19)
  line L7 (12, -19) -> (23.5, -19)
  line L8 (23.5, -19) -> (23.5, -17)
  point P0 (0, -22)
  point P1 (23.5, -19)
  constraints: 16 end point, 4 parallel, 2 horizontal, 2 perpendicular, 1 point on line
extrude "Extrusão25" cut sketch "Esboço27" against normal blind 2
sketch "Esboço28" plane through (0, 22, 0) normal (0, 1, 0) x (1, 0, 0)
  line L0 (-47, 59) -> (-52.5, 59) projected
  line L1 (-2.5, 0) -> (-2.5, 12) projected
  line L2 (-50.5, 59) -> (-4.5, 59)
  line L3 (-2.5, 57) -> (-2.5, 2)
  line L4 (-4.5, 0) -> (-50.5, 0)
  line L5 (-52.5, 2) -> (-52.5, 57)
  arc A0 (-2.5, 57) -> (-4.5, 59) centre (-4.5, 57) ccw
  arc A1 (-4.5, 0) -> (-2.5, 2) centre (-4.5, 2) ccw
  arc A2 (-52.5, 2) -> (-50.5, 0) centre (-50.5, 2) ccw
  arc A3 (-50.5, 59) -> (-52.5, 57) centre (-50.5, 57) ccw
  line L6 (-50.5, 59) -> (-52.5, 59)
  line L7 (-52.5, 59) -> (-52.5, 57)
  line L8 (-4.5, 59) -> (-2.5, 59)
  line L9 (-2.5, 59) -> (-2.5, 57)
  line L10 (-2.5, 2) -> (-2.5, 0)
  line L11 (-4.5, 0) -> (-2.5, 0)
  line L12 (-52.5, 2) -> (-52.5, 0)
  line L13 (-50.5, 0) -> (-52.5, 0)
  line L14 (-52.5, 59) -> (-2.5, 59)
  line L15 (-2.5, 59) -> (-2.5, 59.5243)
  line L16 (-2.5, 59.5243) -> (-52.5, 59.5243)
  line L17 (-52.5, 59.5243) -> (-52.5, 59)
  line L18 (-2.5, 0) -> (-52.5, 0)
  line L19 (-52.5, 0) -> (-52.5, -1)
  line L20 (-52.5, -1) -> (-2.5, -1)
  line L21 (-2.5, -1) -> (-2.5, 0)
  point P0 (0, 0)
  point P1 (-2.5, 2)
  dimension "d132" = 2
  constraints: 40 end point, 13 tangent, 8 point on circle, 8 point on line, 7 perpendicular, 6 parallel, 4 centre point, 3 equal radius, 3 horizontal, 2 collinear
  measures "d132" radius of A0
extrude "Extrusão26" cut sketch "Esboço28" against normal through all contours A3 L7 L0 | L8 L9 A0 | A2 L13 L12 | L1 L11 A1
sketch "Esboço29" plane through (0, 5, 0) normal (0, 1, 0) x (1, 0, 0)
  line L0 (-8, 59) -> (-47, 59) projected
  line L1 (-8, 0) -> (-8, 4) projected
  line L2 (-47, 59) -> (-8, 59)
  line L3 (-8, 59) -> (-8, 0)
  line L4 (-8, 0) -> (-47, 0)
  line L5 (-47, 0) -> (-47, 59)
  point P0 (0, 0)
  constraints: 8 end point, 2 parallel, 1 horizontal, 1 perpendicular
extrude "Extrusão27" cut sketch "Esboço29" against normal blind 1
sketch "Esboço30" plane through (0, 3, 0) normal (0, 1, 0) x (1, 0, 0)
  line L0 (-4.5, 23.5) -> (-21, 23.5) projected
  line L1 (-21, 35.5) -> (-8, 35.5)
  line L2 (-8, 35.5) -> (-8, 23.5)
  line L3 (-8, 23.5) -> (-21, 23.5)
  line L4 (-21, 23.5) -> (-21, 35.5)
  line L5 (-34, 4) -> (-8, 4) projected
  line L6 (-21, 12) -> (-8, 12)
  line L7 (-8, 12) -> (-8, 4)
  line L8 (-8, 4) -> (-21, 4)
  line L9 (-21, 4) -> (-21, 12)
  point P0 (0, 0)
  constraints: 16 end point, 4 parallel, 2 horizontal, 2 perpendicular, 2 point on line
sketch "Esboço31" plane through (0, 3, 0) normal (0, 1, 0) x (1, 0, 0)
  line L0 (-2.5, 35.5) -> (-24, 35.5) projected
  line L1 (-2.5, 4) -> (-2.5, 35.5) projected
  line L2 (-8, 35.5) -> (-2.5, 35.5)
  line L3 (-2.5, 35.5) -> (-2.5, 4)
  line L4 (-2.5, 4) -> (-8, 4)
  line L5 (-8, 4) -> (-8, 35.5)
  point P0 (0, 0)
  constraints: 8 end point, 2 parallel, 1 horizontal, 1 perpendicular, 1 point on line
extrude "Extrusão28" cut sketch "Esboço30" against normal blind 1
sketch "Esboço32" plane through (0, 3, 0) normal (0, 1, 0) x (1, 0, 0)
  point P0 (0, 0)
extrude "Extrusão29" cut sketch "Esboço31" against normal blind 1
sketch "Esboço33" plane through (0, -22, 0) normal (0, -1, 0) x (1, 0, 0)
  line L0 (-24, -15.5) -> (-31, -15.5) projected
  line L1 (-24, -23.5) -> (-31, -23.5) projected
  line L2 (-31, -15.5) -> (-24, -15.5)
  line L3 (-24, -15.5) -> (-24, -23.5)
  line L4 (-24, -23.5) -> (-31, -23.5)
  line L5 (-31, -23.5) -> (-31, -15.5)
  line L6 (-24, -35.5) -> (-31, -35.5) projected
  line L7 (-2.5, -43.5) -> (-52.5, -43.5) projected
  line L8 (-31, -35.5) -> (-24, -35.5)
  line L9 (-24, -35.5) -> (-24, -43.5)
  line L10 (-24, -43.5) -> (-31, -43.5)
  line L11 (-31, -43.5) -> (-31, -35.5)
  point P0 (0, 0)
  constraints: 16 end point, 4 parallel, 2 horizontal, 2 perpendicular, 2 point on line
extrude "Extrusão30" cut sketch "Esboço33" against normal blind 2
sketch "Esboço34" plane through (0, 22, 0) normal (0, 1, 0) x (1, 0, 0)
  line L0 (-47, 59) -> (-50.5, 59) projected
  line L1 (-50.5, 59) -> (-50.5, 47)
  line L2 (-52.5, 57) -> (-52.5, 2) projected
  line L3 (-50.5, 47) -> (-52.5, 47)
  line L4 (-52.5, 47) -> (-52.5, 35.5)
  line L5 (-52.5, 35.5) -> (-50.5, 35.5)
  line L6 (-50.5, 35.5) -> (-50.5, 47)
  point P0 (0, 0)
  dimension "d143" = 11.5
  constraints: 10 end point, 2 parallel, 1 horizontal, 1 perpendicular, 1 point on line, 1 vertical
  measures "d143" distance of L4.end L3.end
extrude "Extrusão31" cut sketch "Esboço34" against normal blind 17
sketch "Esboço35" plane through (0, 3, 0) normal (0, 1, 0) x (1, 0, 0)
  line L0 (-24, 35.5) -> (-31, 35.5) projected
  line L1 (-24, 35.5) -> (-24, 23.5) projected
  line L2 (-31, 35.5) -> (-24, 35.5)
  line L3 (-24, 35.5) -> (-24, 23.5)
  line L4 (-24, 23.5) -> (-31, 23.5)
  line L5 (-31, 23.5) -> (-31, 35.5)
  point P0 (0, 0)
  constraints: 8 end point, 2 parallel, 1 horizontal, 1 perpendicular
extrude "Extrusão32" cut sketch "Esboço35" against normal blind 1
sketch "Esboço36" plane through (0, 4, 0) normal (0, 1, 0) x (1, 0, 0)
  line L0 (-31, 35.5) -> (-52.5, 35.5) projected
  line L1 (-34, 23.5) -> (-52.5, 23.5) projected
  line L2 (-34, 35.5) -> (-47, 35.5)
  line L3 (-47, 35.5) -> (-47, 23.5)
  line L4 (-47, 23.5) -> (-34, 23.5)
  line L5 (-34, 23.5) -> (-34, 35.5)
  point P0 (0, 0)
  constraints: 8 end point, 2 parallel, 2 point on line, 1 horizontal, 1 perpendicular
extrude "Extrusão33" cut sketch "Esboço36" against normal blind 2
sketch "Esboço37" plane through (-52.5, -13, -15.5) normal (-1, 0, 0) x (0, 0, 1)
  line L0 (-31.5, 35) -> (-31.5, 18) projected
  line L1 (-8, 13) -> (-8, 15) projected
  line L2 (-31.5, 18) -> (-8, 18)
  line L3 (-8, 18) -> (-8, 15)
  line L4 (-8, 15) -> (-31.5, 15)
  line L5 (-31.5, 15) -> (-31.5, 18)
  point P0 (15.5, 13)
  constraints: 8 end point, 2 parallel, 1 horizontal, 1 perpendicular
extrude "Extrusão34" cut sketch "Esboço37" against normal blind 2
sketch "Esboço38" plane through (-50.5, 22, -47) normal (-1, 0, 0) x (0, 0, 1)
  line L0 (11.5, -17) -> (23.5, -17) projected
  line L1 (11.5, -20) -> (23.5, -20) projected
  line L2 (11.5, -17) -> (23.5, -17)
  line L3 (23.5, -17) -> (23.5, -20)
  line L4 (23.5, -20) -> (11.5, -20)
  line L5 (11.5, -20) -> (11.5, -17)
  point P0 (47, -22)
  constraints: 8 end point, 2 parallel, 1 horizontal, 1 perpendicular
extrude "Extrusão35" cut sketch "Esboço38" against normal blind 4
sketch "Esboço39" plane through (0, 4, 0) normal (0, 1, 0) x (1, 0, 0)
  line L0 (-21, 35.5) -> (-2.5, 35.5) projected
  line L1 (-8, 59) -> (-10, 59)
  line L2 (-10, 59) -> (-10, 35.5)
  line L3 (-10, 35.5) -> (-8, 35.5)
  line L4 (-8, 35.5) -> (-8, 59)
  point P0 (0, 0)
  constraints: 8 end point, 2 parallel, 1 horizontal, 1 perpendicular, 1 point on line
extrude "Extrusão36" cut sketch "Esboço39" against normal blind 2
sketch "Esboço40" plane through (-21, -12, -12) normal (-1, 0, 0) x (0, 0, 1)
  line L0 (0, 0) -> (0, 2.5)
  line L1 (0, 2.5) -> (8, 2.5)
  line L2 (8, 2.5) -> (8, 7.5)
  line L3 (8, 7.5) -> (0, 7.5)
  line L4 (0, 7.5) -> (0, 2.5)
  point P0 (12, 12)
  dimension "d156" = 2.5
  dimension "d157" = 8
  dimension "d158" = 5
  constraints: 10 end point, 2 parallel, 1 horizontal, 1 perpendicular, 1 vertical
  measures "d156" distance of L0.start L0.end
  measures "d157" distance of L3.end L2.end
  measures "d158" distance of L2.end L1.end
extrude "Extrusão37" cut sketch "Esboço40" against normal blind 2
sketch "Esboço41" plane through (-34, -12, -4) normal (1, 0, 0) x (0, 0, -1)
  line L0 (8, 0) -> (8, 2.5)
  line L1 (0, 0) -> (0, 16) projected
  line L2 (8, 2.5) -> (0, 2.5)
  line L3 (0, 2.5) -> (0, 7.5)
  line L4 (0, 7.5) -> (8, 7.5)
  line L5 (8, 7.5) -> (8, 2.5)
  point P0 (-4, 12)
  dimension "d161" = 2.5
  dimension "d162" = 5
  constraints: 10 end point, 2 parallel, 1 horizontal, 1 perpendicular, 1 point on line, 1 vertical
  measures "d161" distance of L0.start L0.end
  measures "d162" distance of L2.end L3.end
extrude "Extrusão38" cut sketch "Esboço41" against normal blind 2
sketch "Esboço42" plane through (0, -14, 0) normal (0, -1, 0) x (1, 0, 0)
  point P0 (0, 0)
sketch "Esboço43" plane through (0, -14, 0) normal (0, -1, 0) x (1, 0, 0)
  point P0 (0, 0)
sketch "Esboço44" plane through (0, -14, 0) normal (0, -1, 0) x (1, 0, 0)
  line L0 (-2.5, -15.5) -> (-24, -15.5) projected
  line L1 (-52.5, 0) -> (-2.5, 0)
  line L2 (-2.5, 0) -> (-2.5, -15.5)
  line L3 (-2.5, -15.5) -> (-52.5, -15.5)
  line L4 (-52.5, -15.5) -> (-52.5, 0)
  point P0 (0, 0)
  constraints: 8 end point, 2 parallel, 1 horizontal, 1 perpendicular
extrude "Extrusão39" cut sketch "Esboço44" against normal blind 1
sketch "Esboço45" plane through (0, -1, 0) normal (0, -1, 0) x (1, 0, 0)
  line L0 (-52.5, -35.5) -> (-52.5, -43.5) projected
  line L1 (-2.5, -59) -> (-52.5, -59)
  line L2 (-52.5, -59) -> (-52.5, -43.5)
  line L3 (-52.5, -43.5) -> (-2.5, -43.5)
  line L4 (-2.5, -43.5) -> (-2.5, -59)
  point P0 (0, 0)
  constraints: 8 end point, 2 parallel, 1 horizontal, 1 perpendicular
extrude "Extrusão40" cut sketch "Esboço45" against normal blind 1
sketch "Esboço46" plane through (0, -20, 0) normal (0, -1, 0) x (1, 0, 0)
  line L0 (-31, -43.5) -> (-31, -35.5) projected
  line L1 (-31, -35.5) -> (-24, -35.5) projected
  line L2 (-31, -43.5) -> (-29.1, -43.5)
  line L3 (-29.1, -43.5) -> (-29.1, -35.5)
  line L4 (-29.1, -35.5) -> (-31, -35.5)
  line L5 (-31, -35.5) -> (-31, -43.5)
  line L6 (-24, -35.5) -> (-24, -43.5) projected
  line L7 (-24, -43.5) -> (-25.9, -43.5)
  line L8 (-25.9, -43.5) -> (-25.9, -35.5)
  line L9 (-25.9, -35.5) -> (-24, -35.5)
  line L10 (-24, -35.5) -> (-24, -43.5)
  line L11 (-2.5, -15.5) -> (-24, -15.5) projected
  line L12 (-8, -23.5) -> (-47, -23.5) projected
  line L13 (-24, -15.5) -> (-25.9, -15.5)
  line L14 (-25.9, -15.5) -> (-25.9, -23.5)
  line L15 (-25.9, -23.5) -> (-24, -23.5)
  line L16 (-24, -23.5) -> (-24, -15.5)
  line L17 (-31, -23.5) -> (-31, -15.5) projected
  line L18 (-31, -15.5) -> (-29.1, -15.5)
  line L19 (-29.1, -15.5) -> (-29.1, -23.5)
  line L20 (-29.1, -23.5) -> (-31, -23.5)
  line L21 (-31, -23.5) -> (-31, -15.5)
  point P0 (0, 0)
  dimension "d169" = 1.9
  dimension "d170" = 1.9
  dimension "d171" = 1.9
  dimension "d172" = 1.9
  constraints: 32 end point, 8 parallel, 4 horizontal, 4 perpendicular, 4 point on line
  measures "d169" distance of L4.end L3.end
  measures "d170" distance of L8.end L9.end
  measures "d171" distance of L15.end L14.end
  measures "d172" distance of L19.end L20.end
extrude "Extrusão41" cut sketch "Esboço46" against normal blind 14
sketch "Esboço47" plane through (0, -6, 0) normal (0, -1, 0) x (1, 0, 0)
  line L0 (-24, -35.5) -> (-24, -23.5) projected
  line L1 (-25.9, -23.5) -> (-25.9, -15.5) projected
  line L2 (-24, -35.5) -> (-25.9, -35.5)
  line L3 (-25.9, -35.5) -> (-25.9, -23.5)
  line L4 (-25.9, -23.5) -> (-24, -23.5)
  line L5 (-24, -23.5) -> (-24, -35.5)
  line L6 (-31, -23.5) -> (-31, -35.5) projected
  line L7 (-31, -35.5) -> (-29.1, -35.5)
  line L8 (-29.1, -35.5) -> (-29.1, -23.5)
  line L9 (-29.1, -23.5) -> (-31, -23.5)
  line L10 (-31, -23.5) -> (-31, -35.5)
  point P0 (0, 0)
  constraints: 16 end point, 4 parallel, 2 horizontal, 2 perpendicular, 1 point on line
extrude "Extrusão42" cut sketch "Esboço47" against normal blind 14
